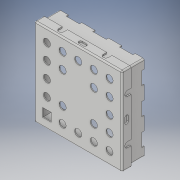
# Autodesk Inventor part: emi_shield
Saved by Autodesk Inventor 2019 (Build 230136000, 136)
## iProperties
Created: 2019-03-13
Part Number: emi_shield
Material: Generico
Document SubType Name: Modeling
Designer: Thartarus
Density: 1 g/cm^3
Appearance: Default
Author: Thartarus
Autodesk Inventor part; units mm, degrees
ref_plane "YZ Plane" through (0, 0, 0) normal (1, 0, 0) x (0, 1, 0)
ref_plane "XZ Plane" through (0, 0, 0) normal (0, 1, 0) x (-1, 0, 0)
ref_plane "XY Plane" through (0, 0, 0) normal (0, 0, 1) x (1, 0, 0)
sketch "Schizzo1" plane through (0, 0, 0) normal (0, 0, 1) x (1, 0, 0)
  line L0 (9.525, -9.525) -> (-9.525, -9.525)
  line L1 (-9.525, -9.525) -> (-9.525, 9.525)
  line L2 (-9.525, 9.525) -> (9.525, 9.525)
  line L3 (9.525, 9.525) -> (9.525, -9.525)
  line L4 (0, 0) -> (15.8702, 0) construction
  line L5 (0, 0) -> (15.8702, 0) construction
  line L6 (9.3218, 9.3218) -> (-9.3218, 9.3218)
  line L7 (-9.3218, 9.3218) -> (-9.3218, -9.3218)
  line L8 (-9.3218, -9.3218) -> (9.3218, -9.3218)
  line L9 (9.3218, -9.3218) -> (9.3218, 9.3218)
  dimension "d0" = 0
  dimension "d1" = 19.05
  dimension "d2" = 0.2032
  constraints: 20 end point, 1 coincident, 1 collinear, 1 horizontal, 1 perpendicular, 12 other
  measures "d0" distance between parallel lines of L4 L5
  measures "d1" distance of L1.end L2.end
  measures "d2" distance between parallel lines of L2 L6
extrude "Estrusione1" add sketch "Schizzo1" along normal blind 5.08
sketch "Schizzo2" plane through (0, 0, 0) normal (0, 0, -1) x (-1, 0, 0)
  line L0 (9.525, -9.525) -> (-9.525, -9.525) projected
  line L1 (9.3218, -9.3218) -> (-9.3218, -9.3218) projected
  line L2 (-7.495, -9.525) -> (-4.5, -9.525)
  line L3 (-4.5, -9.525) -> (-4.5, -9.3218)
  line L4 (-4.5, -9.3218) -> (-7.495, -9.3218)
  line L5 (-7.495, -9.3218) -> (-7.495, -9.525)
  line L6 (-9.525, 9.525) -> (-9.525, -9.525) projected
  line L7 (-1.5, -9.3218) -> (1.5, -9.3218)
  line L8 (1.5, -9.3218) -> (1.5, -9.525)
  line L9 (1.5, -9.525) -> (-1.5, -9.525)
  line L10 (-1.5, -9.525) -> (-1.5, -9.3218)
  line L11 (0, 9.3682) -> (0, 0) construction
  line L12 (4.5, -9.3218) -> (7.495, -9.3218)
  line L13 (7.495, -9.3218) -> (7.495, -9.525)
  line L14 (7.495, -9.525) -> (4.5, -9.525)
  line L15 (4.5, -9.525) -> (4.5, -9.3218)
  line L16 (9.525, -9.525) -> (9.525, 9.525) projected
  line L17 (9.525, 4.5) -> (9.3218, 4.5)
  line L18 (9.3218, 4.5) -> (9.3218, 7.495)
  line L19 (9.3218, 7.495) -> (9.525, 7.495)
  line L20 (9.525, 7.495) -> (9.525, 4.5)
  line L21 (9.3218, 1.5) -> (9.525, 1.5)
  line L22 (9.3218, -1.5) -> (9.3218, 1.5)
  line L23 (9.525, 1.5) -> (9.525, -1.5)
  line L24 (9.525, -1.5) -> (9.3218, -1.5)
  line L25 (9.525, -4.5) -> (9.3218, -4.5)
  line L26 (9.3218, -4.5) -> (9.3218, -7.495)
  line L27 (9.525, -7.495) -> (9.525, -4.5)
  line L28 (9.3218, -7.495) -> (9.525, -7.495)
  line L29 (-4.5, 9.525) -> (-4.5, 9.3218)
  line L30 (-4.5, 9.3218) -> (-7.495, 9.3218)
  line L31 (-7.495, 9.3218) -> (-7.495, 9.525)
  line L32 (-7.495, 9.525) -> (-4.5, 9.525)
  line L33 (-1.5, 9.3218) -> (-1.5, 9.525)
  line L34 (1.5, 9.3218) -> (-1.5, 9.3218)
  line L35 (-1.5, 9.525) -> (1.5, 9.525)
  line L36 (1.5, 9.525) -> (1.5, 9.3218)
  line L37 (4.5, 9.525) -> (4.5, 9.3218)
  line L38 (4.5, 9.3218) -> (7.495, 9.3218)
  line L39 (7.495, 9.525) -> (4.5, 9.525)
  line L40 (7.495, 9.3218) -> (7.495, 9.525)
  line L41 (-9.525, -4.5) -> (-9.3218, -4.5)
  line L42 (-9.3218, -4.5) -> (-9.3218, -7.495)
  line L43 (-9.3218, -7.495) -> (-9.525, -7.495)
  line L44 (-9.525, -7.495) -> (-9.525, -4.5)
  line L45 (-9.3218, -1.5) -> (-9.525, -1.5)
  line L46 (-9.3218, 1.5) -> (-9.3218, -1.5)
  line L47 (-9.525, -1.5) -> (-9.525, 1.5)
  line L48 (-9.525, 1.5) -> (-9.3218, 1.5)
  line L49 (-9.525, 4.5) -> (-9.3218, 4.5)
  line L50 (-9.3218, 4.5) -> (-9.3218, 7.495)
  line L51 (-9.525, 7.495) -> (-9.525, 4.5)
  line L52 (-9.3218, 7.495) -> (-9.525, 7.495)
  dimension "d5" = 2.03
  dimension "d6" = 3
  dimension "d7" = 3
  dimension "d8" = 3
  dimension "d9" = 2.03
  dimension "d12" = 360
  constraints: 98 end point, 6 parallel, 6 point on line, 3 horizontal, 3 perpendicular, 1 vertical, 98 other
  measures "d5" distance between parallel lines of L6 L5
  measures "d6" distance between parallel lines of L8 L10
  measures "d7" distance between parallel lines of L10 L3
  measures "d8" distance between parallel lines of L8 L15
  measures "d9" distance between parallel lines of L16 L13
extrude "Estrusione2" cut sketch "Schizzo2" against normal blind 0.51 contours L0 L15 L1 L13 | L0 L10 L1 L8 | L0 L5 L1 L3 | L52 L50 L49 L6 | L48 L46 L45 L6 | L41 L42 L43 L6 | L28 L26 L25 L16 | L24 L22 L21 L16 | L17 L18 L19 L16 | L29 L30 L31 L32 | L33 L35 L36 L34 | L39 L40 L38 L37
sketch "Schizzo3" plane through (0, 0, 5.08) normal (0, 0, 1) x (1, 0, 0)
  line L0 (-9.83, 9.83) -> (9.83, 9.83)
  line L1 (9.83, 9.83) -> (9.83, -9.83)
  line L2 (9.83, -9.83) -> (-9.83, -9.83)
  line L3 (-9.83, -9.83) -> (-9.83, 9.83)
  line L4 (-9.3218, 9.3218) -> (9.3218, 9.3218) construction
  line L5 (0, 9.3218) -> (0, 0) construction
  line L6 (0, 0) -> (-9.3218, 0) construction
  line L7 (-9.3218, -9.3218) -> (-9.3218, 9.3218) construction
  dimension "d16" = 19.66
  dimension "d17" = 19.66
  constraints: 12 end point, 2 midpoint, 2 parallel, 1 horizontal, 1 perpendicular, 1 vertical, 2 other
  measures "d16" distance of L0.start L0.end
  measures "d17" distance of L0.end L1.end
extrude "Estrusione3" add sketch "Schizzo3" along normal blind 0.2 and the other way blind 1.81
fillet "Raccordo1" radius 0.3 12 edges at (9.525, 9.525, 1.635) (9.83, 9.83, 4.275) (-9.83, 9.83, 4.275) (-9.525, 9.525, 1.635) (0, 9.83, 5.28) (-9.83, 0, 5.28) (9.83, 0, 5.28) (0, -9.83, 5.28) (9.83, -9.83, 4.275) (9.525, -9.525, 1.635) (-9.83, -9.83, 4.275) (-9.525, -9.525, 1.635)
sketch "Schizzo4" plane through (-9.53, 9.83, 4.98) normal (0, 1, 0) x (1, 0, 0)
  line L0 (15.12, 1.71) -> (13.92, 1.71)
  line L1 (13.92, 1.71) -> (13.92, 0.91)
  line L2 (13.92, 0.91) -> (15.12, 0.91) construction
  line L3 (15.12, 0.91) -> (15.12, 1.71)
  circle A0 centre (14.52, 0.91) radius 0.6 construction
  arc A1 (13.92, 0.91) -> (15.12, 0.91) centre (14.52, 0.91) ccw
  line L4 (0, 1.71) -> (19.06, 1.71) projected
  line L5 (19.36, 0) -> (19.36, 1.71) projected
  line L6 (5.14, 1.71) -> (3.94, 1.71)
  line L7 (3.94, 1.71) -> (3.94, 0.91)
  line L8 (3.94, 0.91) -> (5.14, 0.91) construction
  line L9 (5.14, 0.91) -> (5.14, 1.71)
  circle A2 centre (4.54, 0.91) radius 0.6 construction
  arc A3 (3.94, 0.91) -> (5.14, 0.91) centre (4.54, 0.91) ccw
  line L10 (-0.3, 1.71) -> (-0.3, 0) projected
  line L11 (10.025, 0.31) -> (9.035, 0.31)
  line L12 (9.035, 0.31) -> (9.035, 1.1) construction
  line L13 (9.035, 1.1) -> (10.025, 1.1)
  line L14 (10.025, 1.1) -> (10.025, 0.31) construction
  arc A4 (10.025, 0.31) -> (10.025, 1.1) centre (10.025, 0.705) ccw
  arc A5 (9.035, 1.1) -> (9.035, 0.31) centre (9.035, 0.705) ccw
  line L15 (10.025, 0.705) -> (9.035, 0.705) construction
  line L16 (0, -0.3) -> (19.06, -0.3) projected
  point P0 (9.53, 4.98)
  point P1 (14.52, 0.31)
  point P2 (19.36, 1.41)
  point P3 (4.54, 0.31)
  point P4 (9.53, 0.705)
  point P5 (8.64, 0.705)
  point P6 (10.42, 0.705)
  dimension "d23" = 1.2
  dimension "d24" = 1.4
  dimension "d26" = 1.2
  dimension "d27" = 1.4
  dimension "d30" = 4.24
  dimension "d31" = 4.24
  dimension "d32" = 8.94
  dimension "d33" = 8.94
  dimension "d91" = 0.61
  dimension "d92" = 0.61
  constraints: 26 end point, 12 point on circle, 8 tangent, 6 parallel, 4 centre point, 4 horizontal, 3 midpoint, 3 perpendicular, 2 collinear, 2 horizontal alignment, 1 point on line, 4 other
  measures "d23" distance between parallel lines of L1 L3
  measures "d24" distance from line of L0 point (14.52, 0.31)
  measures "d26" distance between parallel lines of L7 L9
  measures "d27" distance from line of L6 point (4.54, 0.31)
  measures "d30" distance between parallel lines of L10 L7
  measures "d31" distance between parallel lines of L5 L3
  measures "d32" distance from line of L10 point (8.64, 0.705)
  measures "d33" distance from line of point (10.42, 0.705) L5
  measures "d91" distance between parallel lines of L16 L11
  measures "d92" distance between parallel lines of L4 L13
extrude "Estrusione4" cut sketch "Schizzo4" against normal up to surface (0.305 mm away)
sketch "Schizzo5" plane through (0, 0, 5.28) normal (0, 0, 1) x (1, 0, 0)
  line L0 (-7.98, -6.05) -> (-6.05, -6.05)
  line L1 (-6.05, -6.05) -> (-6.05, -7.98)
  line L2 (-6.05, -7.98) -> (-7.98, -7.98)
  line L3 (-7.98, -7.98) -> (-7.98, -6.05)
  line L4 (-9.83, 9.53) -> (-9.83, -9.53) projected
  line L5 (-9.53, -9.83) -> (9.53, -9.83) projected
  line L6 (-7.015, -7.015) -> (-7.015, 7.015) construction
  line L7 (-7.015, 7.015) -> (7.015, 7.015) construction
  line L8 (7.015, 7.015) -> (7.015, -7.015) construction
  line L9 (7.015, -7.015) -> (-7.015, -7.015) construction
  circle A0 centre (-7.015, 7.015) radius 0.8
  circle A1 centre (7.015, -7.015) radius 0.8
  circle A2 centre (-7.015, 3.505) radius 0.8
  circle A3 centre (-7.015, -0.005) radius 0.8
  circle A4 centre (-3.505, 7.015) radius 0.8
  circle A5 centre (-3.505, 3.505) radius 0.8
  circle A6 centre (-3.505, -0.005) radius 0.8
  circle A7 centre (0.005, 7.015) radius 0.8
  circle A8 centre (0.005, 3.505) radius 0.8
  circle A9 centre (0.005, -0.005) radius 0.8
  circle A10 centre (-7.015, -3.515) radius 0.8
  circle A11 centre (-3.505, -3.515) radius 0.8
  circle A12 centre (0.005, -3.515) radius 0.8
  circle A13 centre (3.515, 7.015) radius 0.8
  circle A14 centre (3.515, 3.505) radius 0.8
  circle A15 centre (3.515, -0.005) radius 0.8
  circle A16 centre (3.515, -3.515) radius 0.8
  circle A17 centre (7.025, 7.015) radius 0.8
  circle A18 centre (7.025, 3.505) radius 0.8
  circle A19 centre (7.025, -0.005) radius 0.8
  circle A20 centre (7.025, -3.515) radius 0.8
  circle A21 centre (3.505, -7.015) radius 0.8
  circle A22 centre (-0.005, -7.015) radius 0.8
  circle A23 centre (-3.515, -7.015) radius 0.8
  point P0 (0, 0)
  point P1 (0, 0)
  dimension "d38" = 1.93
  dimension "d39" = 1.85
  dimension "d40" = 1.85
  dimension "d41" = 1.6
  dimension "d42" = 1.6
  dimension "d45" = 3.51
  dimension "d48" = 3.51
  dimension "d53" = 3.51
  constraints: 24 centre point, 16 end point, 3 coincident, 2 horizontal, 1 vertical, 62 other
  measures "d38" distance of L1.end L2.end
  measures "d39" distance between parallel lines of L4 L3
  measures "d40" distance between parallel lines of L5 L2
  measures "d41" diameter of A0
  measures "d42" diameter of A1
  measures "d45" distance of A0.centre A2.centre
  measures "d48" distance of A0.centre A4.centre
  measures "d53" distance of A1.centre A21.centre
extrude "Estrusione5" cut sketch "Schizzo5" against normal up to surface (5.28 mm away) contours L0 L1 L2 L3 | A0 | A1 | A2 | A3 | A4 | A5 | A7 | A10 | A11 | A13 | A14 | A16 | A17 | A18 | A19 | A20 | A21 | A22 | A23
sketch "Schizzo6" plane through (0, 0, 3.27) normal (0, 0, -1) x (-1, 0, 0)
  line L0 (-9.3218, 9.3218) -> (-7.495, 9.3218) projected
  line L1 (-9.3218, 9.3218) -> (9.3218, 9.3218)
  line L2 (9.3218, 9.3218) -> (9.3218, -9.3218)
  line L3 (9.3218, -9.3218) -> (-9.3218, -9.3218)
  line L4 (-9.3218, -9.3218) -> (-9.3218, 9.3218)
  line L5 (9.3218, -1.5) -> (9.3218, -4.5) projected
  line L6 (9.3218, -9.3218) -> (7.495, -9.3218) projected
  point P0 (0, 0)
  constraints: 8 end point, 2 collinear, 2 parallel, 1 horizontal, 1 perpendicular
extrude "Estrusione6" cut sketch "Schizzo6" against normal blind 1.81
sketch "Schizzo8" plane through (0, 0, 5.08) normal (0, 0, -1) x (-1, 0, 0)
  circle A0 centre (0, 0) radius 2.995
  dimension "d85" = 5.99
  dimension "d62" = 5.99
  dimension "d63" = 0.99
  dimension "d66" = 360
  dimension "d68" = 0.99
  dimension "d74" = 0.99
  dimension "d76" = 0.99
  dimension "d77" = 0.99
  dimension "d78" = 45
  dimension "d80" = 2.01
  dimension "d83" = 360
  constraints: 1 centre point, 1 coincident
  measures "d85" diameter of A0
extrude "Estrusione7" add sketch "Schizzo8" along normal blind 0.08
pattern_circular "Serie circolare1" count 4 over 360 about axis through (0, 0, 5.08) along (0, 0, -1) of "Estrusione4"
